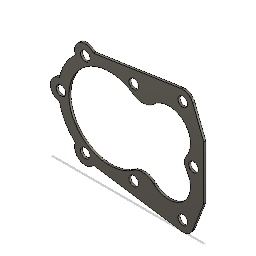
_evaluative 6.15871b31-741a-4c59-b3b1-ab99563532c6 (Autodesk Fusion 360 design; units mm, degrees)
Autodesk Fusion 360 part; units mm, degrees
note: some values were not read from the file. Set by a fixed rule: which sketch regions a step uses.
sketch "Sketch1" plane through (0, 0, 0) normal (0, 0, 1) x (1, 0, 0)
  circle A0 centre (0, 0) radius 45.72 construction
  circle A1 centre (22.86, 39.5947) radius 4.4196
  line L0 (0, 0) -> (0, 63.5) construction
  line L1 (22.86, 39.5947) -> (0, 0) construction
  line L2 (0, 0) -> (69.088, 0) construction
  circle A2 centre (-22.86, 39.5947) radius 4.4196
  circle A3 centre (-45.72, 0) radius 4.4196
  circle A4 centre (-22.86, -39.5947) radius 4.4196
  circle A5 centre (22.86, -39.5947) radius 4.4196
  arc A6 (-14.8961, 45.9035) -> (-32.3056, 35.8522) centre (-22.86, 39.5947) ccw
  arc A7 (-47.2017, 10.0514) -> (-47.2017, -10.0514) centre (-45.72, 0) ccw
  arc A8 (-32.3056, -35.8522) -> (-14.8961, -45.9035) centre (-22.86, -39.5947) ccw
  line L3 (55.88, 55.88) -> (55.88, -43.18) construction
  arc A9 (22.2359, 30.9383) -> (41.7373, 32.3706) centre (31.1302, 43.3136) ccw
  arc A10 (45.7196, 0.1826) -> (46.0426, 0) centre (55.88, 17.78) ccw
  arc A11 (72.3846, 5.9267) -> (41.7373, 32.3706) centre (55.88, 17.78) ccw
  circle A12 centre (69.088, 48.26) radius 4.4196
  line L4 (-14.8961, 45.9035) -> (67.577, 58.307)
  line L5 (88.9, 25.4) -> (88.9, -25.4)
  line L6 (88.9, 25.4) -> (78.5547, 51.9489)
  circle A13 centre (79.248, 0) radius 4.4196
  arc A14 (22.2359, 30.9383) -> (22.2359, -30.9383) centre (0, 0) ccw
  arc A15 (0.7353, 48.2544) -> (0, 48.26) centre (0, 0) ccw
  arc A16 (78.5547, 51.9489) -> (67.577, 58.307) centre (69.088, 48.26) ccw
  line L7 (-14.8961, -45.9035) -> (67.577, -58.307)
  arc A17 (67.577, -58.307) -> (78.5547, -51.9489) centre (69.088, -48.26) ccw
  line L8 (88.9, -25.4) -> (78.5547, -51.9489)
  arc A18 (41.7373, -32.3706) -> (72.3846, -5.9267) centre (55.88, -17.78) ccw
  arc A19 (41.7373, -32.3706) -> (22.2359, -30.9383) centre (31.1302, -43.3136) ccw
  arc A20 (-32.3056, 35.8522) -> (-47.2017, 10.0514) centre (0, 0) ccw
  arc A21 (-47.2017, -10.0514) -> (-32.3056, -35.8522) centre (0, 0) ccw
  circle A22 centre (69.088, -48.26) radius 4.4196
  arc A23 (72.3846, 5.9267) -> (72.3846, -5.9267) centre (80.6369, 0) ccw
  dimension "d2" = 91.44
  dimension "d3" = 76.2
  dimension "d4" = 8.8392
  dimension "d5" = 30
  dimension "d7" = 240
  dimension "d13" = 55.88
  dimension "d14" = 40.64
  dimension "d15" = 17.78
  dimension "d16" = 30.48
  dimension "d17" = 8.8392
  dimension "d18" = 48.26
  dimension "d19" = 69.088
  dimension "d20" = 20.32
  dimension "d21" = 134.62
  dimension "d22" = 25.4
  dimension "d23" = 8.8392
  dimension "d24" = 79.248
  dimension "d28" = 20.32
  measures "d2" diameter of A0
  measures "d3" diameter of A14
  measures "d4" diameter of A1
  measures "d5" angle of L0 L1
  measures "d14" diameter of A10
  measures "d15" distance of A0.centre
  measures "d16" diameter of A9
  measures "d17" diameter of A12
  measures "d20" diameter of A16
  measures "d23" diameter of A13
  measures "d28" diameter of A23
extrude "Extrude1" add sketch "Sketch1" along normal mid plane 2.032
